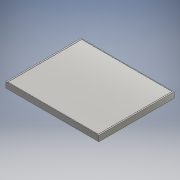
# Autodesk Inventor part: TFT_case
Saved by Autodesk Inventor 2016 (Build 200138000, 138)
## iProperties
Created: 2016-09-20
Part Number: TFT_case
Material: 一般
Document SubType Name: Modeling
Designer: KOTA-NPC2
Density: 1 g/cm^3
Appearance: 機械加工 - アルミニウム
Author: KOTA-NPC2
Autodesk Inventor part; units mm, degrees
ref_plane "YZ Plane" through (0, 0, 0) normal (1, 0, 0) x (0, 1, 0)
ref_plane "XZ Plane" through (0, 0, 0) normal (0, 1, 0) x (-1, 0, 0)
ref_plane "XY Plane" through (0, 0, 0) normal (0, 0, 1) x (1, 0, 0)
sketch "スケッチ1" plane through (0, 0, 0) normal (0, 0, 1) x (1, 0, 0)
  line L0 (-18.25, 14.75) -> (18.25, 14.75)
  line L1 (18.25, 14.75) -> (18.25, -14.75)
  line L2 (18.25, -14.75) -> (-18.25, -14.75)
  line L3 (-18.25, -14.75) -> (-18.25, 14.75)
  line L4 (0, 17.8351) -> (0, -18.1881) construction
  circle A0 centre (0, 7.75) radius 0.5
  circle A1 centre (0, 3.75) radius 0.5
  point P0 (0, 0)
  dimension "d0" = 18.25
  dimension "d1" = 18.25
  dimension "d2" = 14.75
  dimension "d3" = 14.75
  dimension "d18" = 1
  dimension "d19" = 7
  dimension "d20" = 1
  dimension "d21" = 4
  constraints: 10 end point, 2 centre point, 2 parallel, 2 point on line, 1 horizontal, 1 perpendicular, 1 vertical, 2 other
  measures "d0" distance from line of L1 point (0, 0)
  measures "d1" distance from line of point (0, 0) L3
  measures "d2" distance from line of point (0, 0) L0
  measures "d3" distance from line of point (0, 0) L2
  measures "d18" diameter of A0
  measures "d19" distance from line of L0 A0.centre
  measures "d20" diameter of A1
  measures "d21" distance of A1.centre A0.centre
extrude "押し出し1" add sketch "スケッチ1" along normal blind 2.25 contours L0 L1 L2 L3 | A0 | A1
sketch "スケッチ2" plane through (0, 0, 2.25) normal (0, 0, 1) x (1, 0, 0)
  line L0 (-17.75, 14.5) -> (17.75, 14.5)
  line L1 (17.75, 14.5) -> (17.75, -14.5)
  line L2 (17.75, -14.5) -> (-17.75, -14.5)
  line L3 (-17.75, -14.5) -> (-17.75, 14.5)
  line L4 (18.25, -14.75) -> (18.25, 14.75) projected
  point P0 (0, 0)
  dimension "d6" = 0.5
  dimension "d7" = 35.5
  dimension "d8" = 14.5
  dimension "d9" = 14.5
  constraints: 8 end point, 2 parallel, 1 horizontal, 1 perpendicular
  measures "d6" distance between parallel lines of L4 L1
  measures "d7" distance between parallel lines of L3 L1
  measures "d8" distance from line of point (0, 0) L0
  measures "d9" distance from line of point (0, 0) L2
extrude "押し出し2" cut sketch "スケッチ2" against normal blind 0.05
extrude "押し出し5" cut sketch "スケッチ1" along normal blind 1 contours A0 | A1
equation "\"d1\" = d0"
equation "\"d3\" = d2"
equation "\"d9\" = d8"
